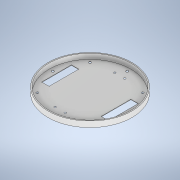
# Autodesk Inventor part: caseBottom
Saved by Autodesk Inventor 2020 (Build 240168000, 168)
## iProperties
Created: 2020-04-07
Part Number: caseBottom
Material: Пластик АБС
Document SubType Name: Modeling
Designer: jamnissa
Density: 1.06 g/cm^3
Appearance: Гладкий — белый
Mass: 15.3017 g
Surface Area: 408.297 cm^2
Volume: 14.4356 cm^3
Author: jamnissa
Autodesk Inventor part; units mm, degrees
ref_plane "YZ Plane" through (0, 0, 0) normal (1, 0, 0) x (0, 1, 0)
ref_plane "XZ Plane" through (0, 0, 0) normal (0, 1, 0) x (-1, 0, 0)
ref_plane "XY Plane" through (0, 0, 0) normal (0, 0, 1) x (1, 0, 0)
sketch "Эскиз1" plane through (0, 0, 0) normal (0, 1, 0) x (-1, 0, 0)
  circle A0 centre (0, 0) radius 56.5
  line L0 (79.4555, 0) -> (-79.4555, 0)
  line L1 (0, -103.8803) -> (0, 88.3129)
  circle A1 centre (0, 0) radius 55
  line L2 (0, -103.8803) -> (0, 88.3129)
  line L3 (-79.4555, 0) -> (79.4555, 0)
  line L4 (11.5, -13.3) -> (23, -13.3)
  line L5 (23, -13.3) -> (23, 13.3)
  line L6 (23, 13.3) -> (11.5, 13.3)
  line L7 (11.5, 13.3) -> (11.5, -13.3)
  line L8 (35, -20) -> (45, -20)
  line L9 (45, -20) -> (45, 20)
  line L10 (45, 20) -> (35, 20)
  line L11 (35, 20) -> (35, -20)
  line L12 (17.25, -13.3) -> (17.25, 13.3)
  circle A2 centre (17.25, -9) radius 1
  circle A3 centre (17.25, 9) radius 1
  line L13 (3, 6) -> (33, 6)
  line L14 (33, 6) -> (33, -6)
  line L15 (33, -6) -> (3, -6)
  line L16 (3, -6) -> (3, 6)
  line L17 (-33, 6) -> (-33, -6)
  line L18 (-3, 6) -> (-33, 6)
  line L19 (-3, -6) -> (-3, 6)
  circle A4 centre (-17.25, 9) radius 1
  line L20 (-23, -13.3) -> (-23, 13.3)
  line L21 (-23, 13.3) -> (-11.5, 13.3)
  line L22 (-11.5, 13.3) -> (-11.5, -13.3)
  line L23 (-17.25, -13.3) -> (-17.25, 13.3)
  line L24 (-35, 20) -> (-35, -20)
  line L25 (-45, -20) -> (-45, 20)
  line L26 (-45, 20) -> (-35, 20)
  circle A5 centre (-17.25, -9) radius 1
  line L27 (-11.5, -13.3) -> (-23, -13.3)
  line L28 (-33, -6) -> (-3, -6)
  line L29 (-35, -20) -> (-45, -20)
  circle A6 centre (0, 0) radius 50
  circle A7 centre (0, -50) radius 1.5
  circle A8 centre (50, 0) radius 1.5
  circle A9 centre (0, 50) radius 1.5
  circle A10 centre (-50, 0) radius 1.5
  circle A11 centre (35.3553, -35.3553) radius 1.5
  circle A12 centre (50, 0) radius 1.5
  circle A13 centre (35.3553, 35.3553) radius 1.5
  circle A14 centre (0, 50) radius 1.5
  circle A15 centre (-35.3553, 35.3553) radius 1.5
  circle A16 centre (-50, 0) radius 1.5
  circle A17 centre (-35.3553, -35.3553) radius 1.5
  dimension "d0" = 113
  dimension "d135" = 11.5
  dimension "d136" = 26.6
  dimension "d137" = 10
  dimension "d138" = 40
  dimension "d139" = 45
  dimension "d140" = 12
  dimension "d141" = 2
  dimension "d142" = 18
  dimension "d143" = 2
  dimension "d144" = 30
  dimension "d145" = 12
  dimension "d146" = 2
  dimension "d147" = 100
  dimension "d148" = 3
  dimension "d149" = 3
  dimension "d150" = 3
  dimension "d151" = 3
  dimension "d152" = 360
  constraints: 60 end point, 18 centre point, 17 symmetric about line, 9 point on line, 6 parallel, 4 horizontal, 4 point on circle, 3 midpoint, 3 perpendicular, 2 coincident, 1 vertical, 22 other
  measures "d0" diameter of A0
  measures "d135" distance of L5.end L6.end
  measures "d136" distance of L4.end L5.end
  measures "d137" distance of L10.end L9.end
  measures "d138" distance of L10.end L8.start
  measures "d139" distance from line of L9 A1.centre
  measures "d140" distance between parallel lines of L11 L5
  measures "d141" diameter of A3
  measures "d142" distance of A3.centre A2.centre
  measures "d143" diameter of A2
  measures "d144" distance of L15.end L14.end
  measures "d145" distance of L15.end L13.start
  measures "d146" distance between parallel lines of L11 L14
  measures "d147" diameter of A6
  measures "d148" diameter of A7
  measures "d149" diameter of A8
  measures "d150" diameter of A9
  measures "d151" diameter of A10
extrude "Выдавливание1" add sketch "Эскиз1" along normal blind 2
sketch "Эскиз2" plane through (0, 0, 0) normal (0, -1, 0) x (1, 0, 0)
  circle A0 centre (0, 0) radius 57
  line L0 (0, -103.8803) -> (0, 88.3129)
  line L1 (-79.4555, 0) -> (79.4555, 0) projected
  circle A1 centre (0, 0) radius 50
  circle A2 centre (0, -50) radius 1.5
  circle A3 centre (50, 0) radius 1.5
  circle A4 centre (0, 50) radius 1.5
  circle A5 centre (-50, 0) radius 1.5
  circle A6 centre (35.3553, -35.3553) radius 1.5
  circle A7 centre (50, 0) radius 1.5
  circle A8 centre (35.3553, 35.3553) radius 1.5
  circle A9 centre (0, 50) radius 1.5
  circle A10 centre (-35.3553, 35.3553) radius 1.5
  circle A11 centre (-50, 0) radius 1.5
  circle A12 centre (-35.3553, -35.3553) radius 1.5
  circle A13 centre (0, 50) radius 2.8
  circle A14 centre (-11, 24) radius 1.5
  circle A15 centre (11, 24) radius 1.5
  circle A16 centre (11, -24) radius 1.5
  circle A17 centre (11, 24) radius 1.5
  circle A18 centre (-11, -24) radius 1.5
  circle A19 centre (-11, 24) radius 1.5
  circle A20 centre (50, 0) radius 1.5
  circle A21 centre (-50, 0) radius 1.5
  circle A22 centre (-17.25, -9) radius 1
  circle A23 centre (-35.3553, -35.3553) radius 1.5
  circle A24 centre (35.3553, 35.3553) radius 1.5
  circle A25 centre (35.3553, -35.3553) radius 1.5
  circle A26 centre (-35.3553, 35.3553) radius 1.5
  circle A27 centre (17.25, -9) radius 1
  circle A28 centre (17.25, 9) radius 1
  circle A29 centre (-17.25, 9) radius 1
  circle A30 centre (0, -50) radius 1.5
  circle A31 centre (0, 50) radius 1.5
  circle A32 centre (0, 0) radius 55
  line L2 (0, 103.8803) -> (0, -88.3129)
  line L3 (-79.4555, 0) -> (79.4555, 0)
  circle A33 centre (6.75, 40) radius 1.15
  circle A34 centre (-6.75, 40) radius 1.15
  circle A35 centre (6.75, -40) radius 1.15
  circle A36 centre (-6.75, -40) radius 1.15
  dimension "d22" = 3
  dimension "d23" = 3
  dimension "d26" = 3
  dimension "d30" = 360
  dimension "d84" = 114
  dimension "d118" = 5.6
  dimension "d155" = 2.3
  dimension "d156" = 13.5
  dimension "d157" = 10
  dimension "d158" = 2.3
  dimension "d159" = 13.5
  dimension "d160" = 10
  constraints: 37 centre point, 6 end point, 4 point on circle, 4 point on line, 2 coincident, 2 symmetric about line, 19 other
  measures "d22" diameter of A2
  measures "d23" diameter of A3
  measures "d26" diameter of A5
  measures "d84" diameter of A0
  measures "d118" diameter of A13
  measures "d155" diameter of A33
  measures "d156" distance of A33.centre A34.centre
  measures "d157" vertical distance of A31.centre A33.centre
  measures "d158" diameter of A35
  measures "d159" distance of A35.centre A36.centre
  measures "d160" vertical distance of A30.centre A35.centre
sketch "Эскиз6" plane through (0, 2, 0) normal (0, 1, 0) x (1, 0, 0)
  circle A0 centre (0, 0) radius 56.5 projected
  dimension "d85" = 113
  measures "d85" diameter of A0
ref_plane "РабПлоскость9" through (0, 52.6, 0) normal (0, 1, 0) x (1, 0, 0)
ref_plane "РабПлоскость11" through (0, 52.6, 0) normal (0, 1, 0) x (1, 0, 0)
sketch "Эскиз8" plane through (0, 52.6, 0) normal (0, 1, 0) x (1, 0, 0)
  circle A0 centre (0, 0) radius 55
  dimension "d83" = 110
  constraints: 1 centre point, 1 coincident
  measures "d83" diameter of A0
extrude "Выдавливание9" cut sketch "Эскиз8" against normal blind 52
ref_plane "РабПлоскость6" through (-79.4555, 0, 0) normal (0, 0, -1) x (1, 0, 0)
ref_plane "РабПлоскость8" through (0, 7.611, 0) normal (0, -1, 0) x (1, 0, 0)
sketch "Эскиз11" plane through (0, 7.611, 0) normal (0, -1, 0) x (1, 0, 0)
  circle A0 centre (0, 0) radius 56.5
  dimension "d108" = 113
  constraints: 1 centre point
  measures "d108" diameter of A0
sketch "Эскиз12" plane through (0, 7.611, 0) normal (0, -1, 0) x (1, 0, 0)
  circle A0 centre (0, 0) radius 55
  dimension "d109" = 110
  constraints: 1 centre point, 1 coincident
  measures "d109" diameter of A0
loft "Лофт2" add profiles "Эскиз11" section 2 edges at (56.5, 2, 0)
extrude "Выдавливание13" cut sketch "Эскиз12" along normal blind 6
extrude "Выдавливание14" cut sketch "Эскиз2" against normal through all contours A2 A1 L0 | L0 A1 A2 | A1 A2 L0 | L0 A2 A1
hole "Отверстие1" at (35.3553, 0, 35.3553) direction (0, 1, 0) diameter 3 end through all countersink diameter 4 countersink angle 90
hole "Отверстие2" at (0, 0, 50) at (-35.3553, 0, 35.3553) at (-50, 0, 0) at (-35.3553, 0, -35.3553) at (0, 0, -50) at (35.3553, 0, -35.3553) at (50, 0, 0) direction (0, 1, 0) diameter 3 end through all countersink diameter 4 countersink angle 90
extrude "Выдавливание15" cut sketch "Эскиз1" along normal through all contours L9 L8 L11 L0 | L0 L11 L10 L9 | L25 L26 L24 L0 | L0 L24 L29 L25
hole "Отверстие3" at (6.75, 0, -40) at (-6.75, 0, -40) at (6.75, 0, 40) at (-6.75, 0, 40) direction (0, 1, 0) diameter 1.567 end through all countersink diameter 3.8 countersink angle 90 thread size "M2x0.4" class "6H" standard "ISO Metric profile"
